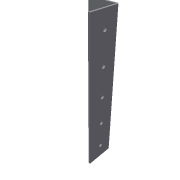
# Autodesk Inventor part: Angle bracket
Saved by Autodesk Inventor 2014 (Build 180170000, 170)
## iProperties
Created: 2014-01-25
Part Number: Angle bracket
Material: Generic
Document SubType Name: Modeling
Designer: elitwack
Density: 1 g/cm^3
Appearance: Default
Author: elitwack
Autodesk Inventor part; units mm, degrees
ref_plane "YZ Plane" through (0, 0, 0) normal (1, 0, 0) x (0, 1, 0)
ref_plane "XZ Plane" through (0, 0, 0) normal (0, 1, 0) x (-1, 0, 0)
ref_plane "XY Plane" through (0, 0, 0) normal (0, 0, 1) x (1, 0, 0)
sketch "Sketch1" plane through (0, 0, 0) normal (0, 0, 1) x (1, 0, 0)
  line L0 (-23.7998, 0) -> (0, 0)
  line L1 (0, 0) -> (0, -127)
  line L2 (0, -127) -> (-23.7998, -127)
  line L3 (-23.7998, -127) -> (-23.7998, 0)
  circle A0 centre (-11.0998, -12.7) radius 1.7859
  circle A1 centre (-11.0998, -38.1) radius 1.7859
  circle A2 centre (-11.0998, -63.5) radius 1.7859
  circle A3 centre (-11.0998, -88.9) radius 1.7859
  circle A4 centre (-11.0998, -114.3) radius 1.7859
  line L4 (-11.0998, -12.7) -> (-11.0998, -38.1) construction
  line L5 (-11.0998, -38.1) -> (-11.0998, -63.5) construction
  line L6 (-11.0998, -63.5) -> (-11.0998, -88.9) construction
  line L7 (-11.0998, -88.9) -> (-11.0998, -114.3) construction
  dimension "d0" = 23.7998
  dimension "d1" = 127
  dimension "d2" = 3.5719
  dimension "d3" = 25.4
  dimension "d4" = 12.7
  dimension "d5" = 11.0998
  constraints: 16 end point, 6 collinear, 5 centre point, 4 equal radius, 3 parallel, 1 coincident, 1 horizontal, 1 perpendicular
  measures "d0" distance of L1.end L2.end
  measures "d1" distance of L0.end L1.end
  measures "d2" diameter of A0
  measures "d3" distance of L4.start L4.end
  measures "d4" distance from line of L0 L4.start
  measures "d5" distance from line of L1 L4.start
extrude "Extrusion1" add sketch "Sketch1" along normal blind 1.5875
sketch "Sketch3" plane through (0, -127, 0) normal (1, 0, 0) x (0, 0, -1)
  line L0 (-25.3873, 127) -> (-1.5875, 127)
  line L1 (-1.5875, 127) -> (-1.5875, 0)
  line L2 (-1.5875, 0) -> (-25.3873, 0)
  line L3 (-25.3873, 0) -> (-25.3873, 127)
  circle A0 centre (-12.6873, 114.3) radius 1.7859
  circle A1 centre (-12.6873, 88.9) radius 1.7859
  circle A2 centre (-12.6873, 63.5) radius 1.7859
  circle A3 centre (-12.6873, 38.1) radius 1.7859
  circle A4 centre (-12.6873, 12.7) radius 1.7859
  line L4 (-12.6873, 114.3) -> (-12.6873, 88.9) construction
  line L5 (-12.6873, 88.9) -> (-12.6873, 63.5) construction
  line L6 (-12.6873, 63.5) -> (-12.6873, 38.1) construction
  line L7 (-12.6873, 38.1) -> (-12.6873, 12.7) construction
  dimension "d8" = 23.7998
  dimension "d9" = 127
  dimension "d10" = 3.5719
  dimension "d11" = 25.4
  dimension "d12" = 12.7
  dimension "d13" = 11.0998
  constraints: 16 end point, 6 collinear, 5 centre point, 4 equal radius, 3 parallel, 1 coincident, 1 horizontal, 1 perpendicular
  measures "d8" distance of L1.end L2.end
  measures "d9" distance of L1.end L0.end
  measures "d10" diameter of A0
  measures "d11" distance of L4.start L4.end
  measures "d12" distance from line of L0 L4.start
  measures "d13" distance from line of L1 L4.start
extrude "Extrusion2" add sketch "Sketch3" along normal blind 1.5875
sketch "Sketch4" plane through (0, -127, 1.5875) normal (0, -1, 0) x (1, 0, 0)
  line L0 (0, 0) -> (1.5875, 0) projected
  line L1 (0, 23.7998) -> (1.5875, 23.7998) projected
  line L2 (1.5875, 0) -> (0, -1.5875)
  line L3 (0, -1.5875) -> (0, 0)
  constraints: 4 end point, 1 perpendicular
extrude "Extrusion3" add sketch "Sketch4" against normal blind 127
body "Solid1"
